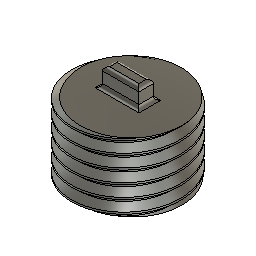
Male Thread Test v2 (Autodesk Fusion 360 design; units mm, degrees)
Autodesk Fusion 360 part; units mm, degrees
sketch "Sketch1" plane through (0, 0, 0) normal (0, 0, 1) x (1, 0, 0)
  circle A0 centre (0, 0) radius 15
  dimension "d1" = 30
  constraint coincident A0.centre origin
  measures "d1" diameter of A0
extrude "Extrude1" add sketch "Sketch1" along normal blind 20
thread "Thread1" "ISO Metric profile 30.0 M30x3.5 6g" major diameter 29.7345 minor diameter 25.732 pitch 3.5 angle 60 modelled right hand crest width 0.4992 on face at (14.9814, -0.7477, 13.3333) crest through (14.8673, 0, -0.875)
sketch "Sketch2" plane through (0, 0, 20) normal (0, 0, 1) x (-1, 0, 0)
  line L0 (5, -2) -> (-5, -2)
  line L1 (-5, -2) -> (-5, 2)
  line L2 (-5, 2) -> (5, 2)
  line L3 (5, 2) -> (5, -2)
  spline S0 degree 3 poles (-14.497, -3.2975) (-13.9541, -5.127) (-13.0634, -6.8343) (-10.701, -9.7681) (-9.2665, -10.9777) (-6.0525, -12.7478) (-4.3131, -13.3072) (-0.7647, -13.7133) (1.0078, -13.5743) (3.8191, -12.7795) (4.8899, -12.3193) (6.8633, -11.1399) (7.7602, -10.4307) (8.5518, -9.6125) knots 0 0 0 0 0.572495 0.572495 1.130652 1.130652 1.674465 1.674465 2.203926 2.203926 2.552907 2.552907 2.895334 2.895334 2.895334 2.895334
  arc A0 (8.5518, -9.6125) -> (11.8756, 4.9501) centre (0, 0) ccw
  spline S1 degree 3 poles (11.8756, 4.9501) (11.3425, 6.5584) (10.4963, 8.0453) (8.2564, 10.6543) (6.8704, 11.7391) (3.7208, 13.3469) (1.9794, 13.8379) (-1.6421, 14.1378) (-3.4885, 13.9255) (-6.4561, 12.9856) (-7.6114, 12.4423) (-9.7702, 11.0581) (-10.7611, 10.2184) (-11.6306, 9.2609) knots 0 0 0 0 0.508319 0.508319 1.030956 1.030956 1.567907 1.567907 2.119164 2.119164 2.499584 2.499584 2.886551 2.886551 2.886551 2.886551
  arc A1 (-11.6306, 9.2609) -> (-14.497, -3.2975) centre (0, 0) ccw
  constraint horizontal L0
  constraint perpendicular L0 L1
  constraint perpendicular L1 L2
  constraint perpendicular L0 L3
extrude "Extrude2" add sketch "Sketch2" along normal blind 5 contours L0 L1 L2 L3
sketch "Sketch3" plane through (0, 0, 0) normal (0, 1, 0) x (1, 0, 0)
fillet "Fillet1" radius 1 4 edges at (0, -2, 20) (5, 0, 20) (0, 2, 20) (-5, 0, 20)
fillet "Fillet2" radius 1 4 edges at (0, 2, 25) (-5, 0, 25) (0, -2, 25) (5, 0, 25)
